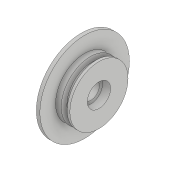
# Autodesk Inventor part: Reel1ACABARMEDIDAS
Saved by Autodesk Inventor 2022 (Build 260153000, 153)
## iProperties
Created: 2019-08-23
Part Number: Reel1ACABARMEDIDAS
Material: Genérico
Document SubType Name: Modeling
Designer: Cristiano
Density: 1 g/cm^3
Appearance: Valor por defecto
Author: Cristiano
Autodesk Inventor part; units mm, degrees
ref_plane "YZ Plane" through (0, 0, 0) normal (1, 0, 0) x (0, 1, 0)
ref_plane "XZ Plane" through (0, 0, 0) normal (0, 1, 0) x (-1, 0, 0)
ref_plane "XY Plane" through (0, 0, 0) normal (0, 0, 1) x (1, 0, 0)
sketch "Boceto1" plane through (0, 0, 0) normal (0, 0, 1) x (1, 0, 0)
  line L0 (0, 0) -> (24.2042, 0) construction
  line L1 (0, 9.5) -> (11, 9.5)
  line L2 (0, 9.5) -> (0, 50)
  line L3 (0, 50) -> (4, 50)
  line L4 (4, 50) -> (4, 32.5)
  line L5 (4, 32.5) -> (10.3205, 32.5)
  line L6 (10.3205, 32.5) -> (11.6603, 27.5)
  line L7 (11.6603, 27.5) -> (15.6603, 27.5)
  line L8 (15.6603, 27.5) -> (17, 32.5)
  line L9 (17, 32.5) -> (20, 32.5)
  line L10 (20, 32.5) -> (20, 13.925)
  line L11 (20, 13.925) -> (11, 13.925)
  line L12 (11, 13.925) -> (11, 9.5)
  line L13 (0, 0) -> (0, 63.5344) construction
  line L14 (13.6603, 27.5) -> (13.6603, 32.5) construction
  line L15 (13.6603, 32.5) -> (10.3205, 32.5) construction
  dimension "d0" = 50
  dimension "d1" = 4
  dimension "d3" = 3
  dimension "d4" = 13.925
  dimension "d5" = 5
  dimension "d6" = 4
  dimension "d7" = 15
  dimension "d8" = 15
  dimension "d10" = 9.5
  dimension "d11" = 9
  dimension "d12" = 32.5
  dimension "d13" = 20
  constraints: 32 end point, 7 perpendicular, 3 vertical, 2 horizontal, 2 point on line, 1 collinear, 1 midpoint, 1 parallel
  measures "d0" distance between parallel lines of L0 L3
  measures "d1" distance of L2.end L3.end
  measures "d3" distance of L8.end L9.end
  measures "d4" distance between parallel lines of L0 L11
  measures "d5" vertical distance of L6.end L5.end
  measures "d6" distance of L6.end L7.end
  measures "d7" angle of L14 L6
  measures "d8" angle of L8 L14
  measures "d10" distance between parallel lines of L0 L1
  measures "d11" distance of L10.end L11.end
  measures "d12" distance between parallel lines of L0 L9
  measures "d13" distance between parallel lines of L2 L10
revolve "Revolución1" add sketch "Boceto1" angle 360 about axis through (0, 0, 0) along (1, 0, 0)
sketch "Sketch2" plane through (20, 0, 0) normal (1, 0, 0) x (0, 0, -1)
  circle A0 centre (0, 0) radius 13.925 projected
  circle A1 centre (0, 0) radius 13
  circle A2 centre (0, 0) radius 13.925 projected
  dimension "d14" = 26
  constraints: 1 centre point, 1 coincident
  measures "d14" diameter of A1
extrude "Extrusion1" add sketch "Sketch2" against normal up to surface (9 mm away)
